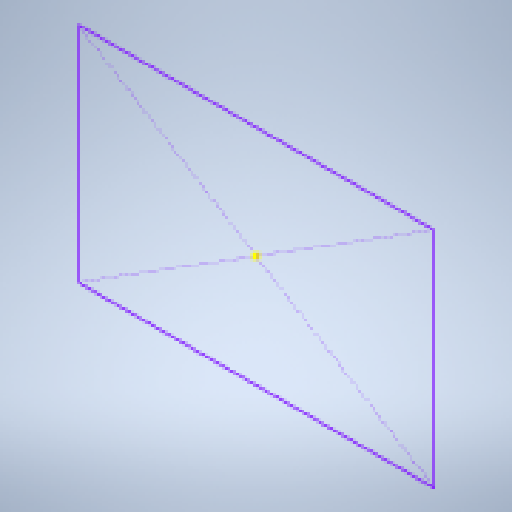
# Autodesk Inventor part: FrameBase
Saved by Autodesk Inventor 2024 (Build 280153000, 153)
## iProperties
Created: 2024-09-07
Part Number: FrameBase
Material: Generic
Document SubType Name: Sheet Metal
Designer: Tommy Rohmann
Density: 1 g/cm^3
Sheet Metal Rule: Default
Appearance: Default
Author: Tommy Rohmann
Autodesk Inventor part; units mm, degrees
ref_plane "YZ Plane" through (0, 0, 0) normal (1, 0, 0) x (0, 1, 0)
ref_plane "XZ Plane" through (0, 0, 0) normal (0, 1, 0) x (-1, 0, 0)
ref_plane "XY Plane" through (0, 0, 0) normal (0, 0, 1) x (1, 0, 0)
sketch "Sketch1" plane through (0, 0, 0) normal (0, 0, 1) x (1, 0, 0)
  line L0 (133.35, -107.95) -> (-133.35, -107.95)
  line L1 (-133.35, -107.95) -> (-133.35, 107.95)
  line L2 (-133.35, 107.95) -> (133.35, 107.95)
  line L3 (133.35, 107.95) -> (133.35, -107.95)
  line L4 (133.35, -107.95) -> (-133.35, 107.95) construction
  line L5 (-133.35, -107.95) -> (133.35, 107.95) construction
  point P0 (0, 0)
  dimension "d0" = 266.7
  dimension "d1" = 215.9
  measures "d0" distance of L1.end L2.end
  measures "d1" distance of L0.end L1.end
extrude "Plate1" add sketch "Sketch1" along normal blind 3.048
equation "\"d0\" = MachineMaxLength"
equation "\"d1\" = MachineMaxWidth"
equation "\"d2\" = Thickness"
equation "\"BendRadius\" = Thickness"
equation "\"BendReliefWidth\" = Thickness"
equation "\"BendReliefDepth\" = 0.5 * Thickness"
equation "\"CornerReliefSize\" = 4 * Thickness"
equation "\"MinimumRemnant\" = 2 * Thickness"
equation "\"TransitionRadius\" = BendRadius"
equation "\"JacobiRadiusSize\" = BendRadius"
equation "\"GapSize\" = Thickness"
equation "\"MachineMaxHeight\" = 539.75"
equation "\"MachineMaxWidth\" = 215.9"
equation "\"MachineMaxLength\" = 266.7"
equation "\"MachineFluidCapacity\" = 25.4"
equation "\"MaxCompressiveCapacity\" = 20320"
equation "\"Thickness\" = 3.048"
body "Solid1"
